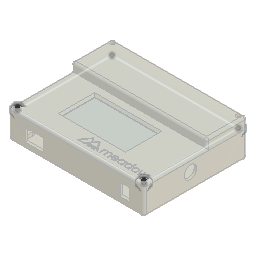
GNSS_Tracker_Enclosure (Autodesk Fusion 360 design; units mm, degrees)
Autodesk Fusion 360 part; units mm, degrees
(part 1 of 4)
sketch "Sketch1" plane through (0, 0, 0) normal (0, 0, 1) x (1, 0, 0) in component "GNSS_PCB"
  line L0 (50, 37.5) -> (-50, 37.5)
  line L1 (-50, 37.5) -> (-50, -37.5)
  line L2 (-50, -37.5) -> (50, -37.5)
  line L3 (50, -37.5) -> (50, 37.5)
  line L4 (50, 37.5) -> (-50, -37.5) construction
  line L5 (-50, 37.5) -> (50, -37.5) construction
  line L6 (0, 37.5) -> (0, -37.5) construction
  line L7 (-50, 0) -> (50, 0) construction
  line L8 (-30.5, 8.425) -> (30.5, 8.425)
  line L9 (30.5, 8.425) -> (30.5, -31.075)
  line L10 (30.5, -31.075) -> (-30.5, -31.075)
  line L11 (-30.5, -31.075) -> (-30.5, 8.425)
  line L12 (-27.5, 1.425) -> (22, 1.425)
  line L13 (22, 1.425) -> (22, -24.075)
  line L14 (22, -24.075) -> (-27.5, -24.075)
  line L15 (-27.5, -24.075) -> (-27.5, 1.425)
  line L16 (-38.5, 35.825) -> (38.5, 35.825)
  line L17 (38.5, 35.825) -> (38.5, 15.175)
  line L18 (38.5, 15.175) -> (-38.5, 15.175)
  line L19 (-38.5, 15.175) -> (-38.5, 35.825)
  line L20 (-33, -37.5) -> (-33, 37.5) construction
  line L21 (38, -37.5) -> (38, 37.5) construction
  line L22 (-28.5, -30.1) -> (-37.5, -30.1)
  line L23 (-37.5, -30.1) -> (-37.5, -37.5)
  line L24 (-37.5, -37.5) -> (-28.5, -37.5)
  line L25 (-28.5, -37.5) -> (-28.5, -30.1)
  line L26 (-28.5, -30.1) -> (-37.5, -37.5) construction
  line L27 (-37.5, -30.1) -> (-28.5, -37.5) construction
  line L28 (40.75, -28.5) -> (35.25, -28.5)
  line L29 (35.25, -28.5) -> (35.25, -40.5)
  line L30 (35.25, -40.5) -> (40.75, -40.5)
  line L31 (40.75, -40.5) -> (40.75, -28.5)
  line L32 (40.75, -28.5) -> (35.25, -40.5) construction
  line L33 (35.25, -28.5) -> (40.75, -40.5) construction
  line L34 (50, -4) -> (-50, -4) construction
  line L35 (-30.5, 3.275) -> (30.5, 3.275)
  line L36 (30.5, 3.275) -> (30.5, -25.925)
  line L37 (30.5, -25.925) -> (-30.5, -25.925)
  line L38 (-30.5, -25.925) -> (-30.5, 3.275)
  line L39 (-50, 35) -> (50, 35) construction
  line L40 (47.5, 37.5) -> (47.5, -37.5) construction
  line L41 (50, -35) -> (-50, -35) construction
  line L42 (-47.5, 37.5) -> (-47.5, -37.5) construction
  line L43 (45, 37.5) -> (45, -37.5) construction
  line L44 (-50, -32.5) -> (50, -32.5) construction
  line L45 (-50, 32.5) -> (50, 32.5) construction
  line L46 (-45, 37.5) -> (-45, -37.5) construction
  line L47 (-50, 30) -> (50, 30) construction
  line L48 (42.5, 37.5) -> (42.5, -37.5) construction
  line L49 (-50, -30) -> (50, -30) construction
  line L50 (-42.5, 37.5) -> (-42.5, -37.5) construction
  arc A0 (-50, -30) -> (-47.5, -32.5) centre (-47.5, -30) ccw
  arc A1 (-45, -35) -> (-47.5, -32.5) centre (-47.5, -35) ccw
  arc A2 (-45, -35) -> (-42.5, -37.5) centre (-42.5, -35) ccw
  arc A3 (47.5, -32.5) -> (50, -30) centre (47.5, -30) ccw
  arc A4 (47.5, -32.5) -> (45, -35) centre (47.5, -35) ccw
  arc A5 (42.5, -37.5) -> (45, -35) centre (42.5, -35) ccw
  arc A6 (50, 30) -> (47.5, 32.5) centre (47.5, 30) ccw
  arc A7 (45, 35) -> (47.5, 32.5) centre (47.5, 35) ccw
  arc A8 (45, 35) -> (42.5, 37.5) centre (42.5, 35) ccw
  arc A9 (-42.5, 37.5) -> (-45, 35) centre (-42.5, 35) ccw
  arc A10 (-47.5, 32.5) -> (-45, 35) centre (-47.5, 35) ccw
  arc A11 (-47.5, 32.5) -> (-50, 30) centre (-47.5, 30) ccw
  point P0 (-33, -33.8)
  point P1 (38, -34.5)
  point P2 (42.5, 35)
  point P3 (47.5, 30)
  point P4 (47.5, 35)
  point P5 (47.5, -30)
  point P6 (42.5, -35)
  point P7 (47.5, -35)
  point P8 (-47.5, 35)
  point P9 (-47.5, 30)
  point P10 (-42.5, 35)
  point P11 (-47.5, -35)
  point P12 (-47.5, -30)
  point P13 (-42.5, -35)
  point P14 (-50, -30)
  point P15 (-47.5, -32.5)
  point P16 (-45, -35)
  point P17 (-42.5, -37.5)
  dimension "d6" = 75
  dimension "d8" = 100
  dimension "d19" = 61
  dimension "d20" = 39.5
  dimension "d21" = 30.5
  dimension "d22" = 8.425
  dimension "d23" = 49.5
  dimension "d24" = 25.5
  dimension "d25" = 7
  dimension "d26" = 3
  dimension "d30" = 77
  dimension "d31" = 20.65
  dimension "d32" = 38.5
  dimension "d35" = 35.825
  dimension "d38" = 17
  dimension "d39" = 12
  dimension "d43" = 9
  dimension "d44" = 7.4
  dimension "d45" = 7.4
  dimension "d49" = 5.5
  dimension "d50" = 12
  dimension "d51" = 9
  dimension "d74" = 61
  dimension "d75" = 29.2
  dimension "d76" = 5.15
  dimension "d167" = 2.5
  dimension "d168" = 2.5
  dimension "d169" = 2.5
  dimension "d170" = 2.5
  dimension "d171" = 2.5
  dimension "d172" = 2.5
  dimension "d173" = 2.5
  dimension "d174" = 2.5
  dimension "d175" = 2.5
  dimension "d176" = 2.5
  dimension "d177" = 2.5
  dimension "d178" = 2.5
  constraint horizontal L0
  constraint perpendicular L0 L1
  constraint parallel L0 L2
  constraint parallel L1 L3
  constraint coincident L4 origin
  constraint coincident L5 origin
  constraint midpoint L0 L6.start
  constraint midpoint L2 L6.end
  constraint midpoint L1 L7.start
  constraint midpoint L3 L7.end
  constraint horizontal L8
  constraint vertical L9
  constraint horizontal L10
  constraint vertical L11
  constraint horizontal L12
  constraint vertical L13
  constraint horizontal L14
  constraint vertical L15
  constraint horizontal L16
  constraint vertical L17
  constraint horizontal L18
  constraint vertical L19
  constraint coincident L2 L20.start
  constraint coincident L0 L20.end
  constraint perpendicular L0 L20
  constraint coincident L2 L21.start
  constraint coincident L0 L21.end
  constraint perpendicular L0 L21
  constraint horizontal L22
  constraint perpendicular L22 L23
  constraint parallel L22 L24
  constraint parallel L23 L25
  constraint coincident L26 P0
  constraint coincident L27 P0
  constraint coincident L20 P0
  constraint horizontal L28
  constraint perpendicular L28 L29
  constraint parallel L28 L30
  constraint parallel L29 L31
  constraint coincident L32 P1
  constraint coincident L33 P1
  constraint coincident L21 P1
  constraint coincident L3 L34.start
  constraint coincident L1 L34.end
  constraint perpendicular L1 L34
  constraint horizontal L35
  constraint vertical L36
  constraint horizontal L37
  constraint vertical L38
  constraint coincident L11 L35.start
  constraint coincident L1 L39.start
  constraint coincident L3 L39.end
  constraint perpendicular L3 L39
  constraint coincident L0 L40.start
  constraint coincident L2 L40.end
  constraint perpendicular L2 L40
  constraint coincident L3 L41.start
  constraint coincident L1 L41.end
  constraint perpendicular L1 L41
  constraint coincident L0 L42.start
  constraint coincident L2 L42.end
  constraint perpendicular L2 L42
  constraint coincident L0 L43.start
  constraint coincident L2 L43.end
  constraint perpendicular L2 L43
  constraint coincident L1 L44.start
  constraint coincident L3 L44.end
  constraint perpendicular L3 L44
  constraint coincident L1 L45.start
  constraint coincident L3 L45.end
  constraint perpendicular L3 L45
  constraint coincident L0 L46.start
  constraint coincident L2 L46.end
  constraint perpendicular L2 L46
  constraint coincident L1 L47.start
  constraint coincident L3 L47.end
  constraint perpendicular L3 L47
  constraint coincident L0 L48.start
  constraint coincident L2 L48.end
  constraint perpendicular L2 L48
  constraint coincident L1 P14
  constraint coincident L3 L49.end
  constraint perpendicular L3 L49
  constraint coincident L0 L50.start
  constraint coincident L2 P17
  constraint perpendicular L2 L50
  constraint coincident L48 P2
  constraint coincident L39 P2
  constraint coincident L47 P3
  constraint coincident L40 P3
  constraint coincident L40 P4
  constraint coincident L39 P4
  constraint coincident L49 P5
  constraint coincident L40 P5
  constraint coincident L48 P6
  constraint coincident L41 P6
  constraint coincident L41 P7
  constraint coincident L40 P7
  constraint coincident L42 P8
  constraint coincident L39 P8
  constraint coincident L47 P9
  constraint coincident L42 P9
  constraint coincident L50 P10
  constraint coincident L39 P10
  constraint coincident L41 P11
  constraint coincident L42 P11
  constraint coincident L42 P12
  constraint coincident L49 P12
  constraint coincident L41 P13
  constraint coincident L50 P13
  constraint coincident P14 L49.start
  constraint coincident L42 P15
  constraint coincident L44 P15
  constraint coincident L46 P16
  constraint coincident L41 P16
  constraint coincident P17 L50.end
  constraint coincident P15 A0.end
  constraint coincident P16 A1.start
  constraint coincident L44 A3.start
  constraint coincident P5 A3.centre
  constraint coincident L43 A4.end
  constraint coincident P7 A4.centre
  constraint coincident L40 A6.end
  constraint coincident P3 A6.centre
  constraint coincident L43 A7.start
  constraint coincident P4 A7.centre
  constraint coincident L46 A9.end
  constraint coincident P10 A9.centre
  constraint coincident L45 A10.start
  constraint coincident P8 A10.centre
  measures "d6" distance of L0.end L1.end
  measures "d8" distance of L0.start L0.end
  measures "d19" distance of L8.start L8.end
  measures "d20" distance of L8.start L10.end
  measures "d21" distance of L6 L11
  measures "d22" distance of L7 L8
  measures "d23" distance of L12.start L12.end
  measures "d24" distance of L12.start L14.end
  measures "d25" distance of L8 L12
  measures "d26" distance of L11 L15
  measures "d30" distance of L16.start L16.end
  measures "d31" distance of L16.start L18.end
  measures "d32" distance of L6 L19
  measures "d35" distance of L7 L16
  measures "d38" distance of L1 L20
  measures "d39" distance of L3 L21
  measures "d43" distance of L23.end L24.end
  measures "d44" distance of L22.end L23.end
  measures "d45" distance of L2 L22
  measures "d49" distance of L29.end L30.end
  measures "d50" distance of L28.end L29.end
  measures "d51" distance of L2 L28
  measures "d74" distance of L35.start L35.end
  measures "d75" distance of L35.start L37.end
  measures "d76" distance of L8 L35
  measures "d167" distance of L0 L39
  measures "d168" distance of L3 L40
  measures "d169" distance of L1 L42
  measures "d170" distance of L2 L41
  measures "d171" distance of L42 L46
  measures "d172" distance of L39 L45
  measures "d173" distance of L40 L43
  measures "d174" distance of L41 L44
  measures "d175" distance of L43 L48
  measures "d176" distance of L45 L47
  measures "d177" distance of L44 L49
  measures "d178" distance of L46 L50
extrude "Extrude1" add sketch "Sketch1" along normal blind 1.7 contours L0 L1 L2 L3 L8 L9 L10 L11 L22 L23 L25 L28 L29 L31 L36 L38 A0 A1 A2 A3 A4 A5 A6 A7 A8 A9 A10 A11 | L2 L28 L29 L31 | L2 L10 L11 L22 L23 L24 L25 | L9 L10 L11 L22 L25 L37 | L10 L11 L22 L25 | L9 L11 L35 L36 L37 L38 | L8 L9 L11 L35 | L12 L13 L14 L15 | L16 L17 L18 L19 makes body 1 in component "GNSS_PCB"
sketch "Sketch2" plane through (0, 0, 1.7) normal (0, 0, 1) x (-1, 0, 0) in component "GNSS_PCB"
  line L0 (42.5, 37.5) -> (-42.5, 37.5)
  line L1 (-50, 30) -> (-50, -30)
  line L2 (-42.5, -37.5) -> (42.5, -37.5)
  line L3 (50, -30) -> (50, 30)
  line L4 (-35.25, 40.5) -> (-40.75, 40.5)
  line L5 (-35.25, 28.5) -> (-35.25, 40.5)
  line L6 (-40.75, 40.5) -> (-40.75, 28.5)
  line L7 (-38, 37.5) -> (-38, -37.5)
  line L8 (-38.5, -15.175) -> (38.5, -15.175)
  line L9 (-38.5, -35.825) -> (-38.5, -15.175)
  line L10 (38.5, -15.175) -> (38.5, -35.825)
  line L11 (38.5, -35.825) -> (-38.5, -35.825)
  line L12 (-40.75, 28.5) -> (-35.25, 28.5)
  arc A0 (-45, -35) -> (-42.5, -37.5) centre (-42.5, -35) ccw
  arc A1 (42.5, -37.5) -> (45, -35) centre (42.5, -35) ccw
  arc A2 (47.5, -32.5) -> (45, -35) centre (47.5, -35) ccw
  arc A3 (47.5, -32.5) -> (50, -30) centre (47.5, -30) ccw
  arc A4 (50, 30) -> (47.5, 32.5) centre (47.5, 30) ccw
  arc A5 (45, 35) -> (47.5, 32.5) centre (47.5, 35) ccw
  arc A6 (45, 35) -> (42.5, 37.5) centre (42.5, 35) ccw
  arc A7 (-42.5, 37.5) -> (-45, 35) centre (-42.5, 35) ccw
  arc A8 (-47.5, 32.5) -> (-45, 35) centre (-47.5, 35) ccw
  arc A9 (-47.5, 32.5) -> (-50, 30) centre (-47.5, 30) ccw
  arc A10 (-50, -30) -> (-47.5, -32.5) centre (-47.5, -30) ccw
  arc A11 (-45, -35) -> (-47.5, -32.5) centre (-47.5, -35) ccw
extrude "Extrude2" add sketch "Sketch2" along normal blind 18.5 separate body contours L7 L8 L10 L11 | L7 L8 L9 L11 makes body 2 in component "GNSS_PCB"
extrude "Extrude3" add sketch "Sketch2" along normal blind 7.5 separate body contours L0 L5 L7 L12 | L0 L4 L5 L6 | L0 L6 L7 L12 makes body 3 in component "GNSS_PCB"
fillet "Fillet1" radius 10.325 1 edges at (0, 15.175, 20.2) on bodies 2 in component "GNSS_PCB"
fillet "Fillet2" radius 10.325 1 edges at (0, 35.825, 20.2) on bodies 2 in component "GNSS_PCB"
ref_plane "WorkPlane1" through (36.625, -33, 3.6) normal (0, 0, 1) x (-1, 0, 0) in component "GNSS_PCB"
sketch "Sketch3" plane through (0, 0, 3.6) normal (0, 0, 1) x (1, 0, 0) in component "GNSS_PCB"
  line L0 (-28.5, -30.1) -> (-37.5, -30.1)
  line L1 (-37.5, -30.1) -> (-37.5, -37.5)
  line L2 (-28.5, -37.5) -> (-28.5, -30.1)
  line L3 (-50, -37.5) -> (50, -37.5)
extrude "Extrude4" add sketch "Sketch3" along normal blind 3.4 separate body makes body 4 in component "GNSS_PCB"
ref_plane "WorkPlane2" through (0, 0, 12.7) normal (0, 0, 1) x (-1, 0, 0) in component "GNSS_PCB"
sketch "Sketch4" plane through (0, 0, 12.7) normal (0, 0, 1) x (1, 0, 0) in component "GNSS_PCB"
  line L0 (-30.5, 8.425) -> (30.5, 8.425)
  line L1 (-30.5, -31.075) -> (-30.5, 8.425)
  line L2 (30.5, 8.425) -> (30.5, -31.075)
  line L3 (30.5, -31.075) -> (-30.5, -31.075)
extrude "Extrude5" add sketch "Sketch4" along normal blind 1.7 separate body makes body 5 in component "GNSS_PCB"
sketch "Sketch5" plane through (0, 0, 14.4) normal (0, 0, 1) x (-1, 0, 0) in component "GNSS_PCB"
  line L0 (-30.5, 31.075) -> (-30.5, -8.425)
  line L1 (-30.5, -8.425) -> (30.5, -8.425)
  line L2 (30.5, -8.425) -> (30.5, 31.075)
  line L3 (30.5, 31.075) -> (-30.5, 31.075)
sketch "Sketch6" plane through (0, 0, 14.4) normal (0, 0, 1) x (-1, 0, 0) in component "GNSS_PCB"
  line L0 (30.5, -3.275) -> (-30.5, -3.275)
  line L1 (-30.5, 25.925) -> (30.5, 25.925)
  line L2 (30.5, 25.925) -> (30.5, -3.275)
  line L3 (-30.5, -3.275) -> (-30.5, 25.925)
extrude "Extrude6" add sketch "Sketch6" along normal blind 1.3 separate body makes body 6 in component "GNSS_PCB"
sketch "Sketch7" plane through (0, 0, 15.7) normal (0, 0, 1) x (-1, 0, 0) in component "GNSS_PCB"
  line L0 (-30.5, -3.275) -> (30.5, -3.275)
  line L1 (30.5, -3.275) -> (30.5, 25.925)
  line L2 (30.5, 25.925) -> (-30.5, 25.925)
  line L3 (-30.5, 25.925) -> (-30.5, -3.275)
  line L4 (-22, 24.075) -> (27.5, 24.075)
  line L5 (-22, -1.425) -> (-22, 24.075)
  line L6 (27.5, 24.075) -> (27.5, -1.425)
  line L7 (27.5, -1.425) -> (-22, -1.425)
hole "Hole1" at (47.5, 30, 1.7) at (47.5, -30, 1.7) at (-47.5, 30, 1.7) at (-47.5, -30, 1.7) direction (0, 0, -1) diameter 2.1 end through all bodies 1 2 3 in component "GNSS_PCB"
ref_plane "WorkPlane1" through (0, 0, -3) normal (0, 0, 1) x (1, 0, 0) in component "GNSS_Enclosure_Bottom"
sketch "Sketch1 (2)" plane through (0, 0, -3) normal (0, 0, 1) x (1, 0, 0) in component "GNSS_Enclosure_Bottom"
  line L0 (-50, -37.5) -> (50, -37.5)
  line L1 (50, -37.5) -> (50, 37.5)
  line L2 (50, 37.5) -> (-50, 37.5)
  line L3 (-50, 37.5) -> (-50, -37.5)
  line L4 (51, -38.5) -> (51, 38.5)
  line L5 (51, 38.5) -> (-51, 38.5)
  line L6 (-51, 38.5) -> (-51, -38.5)
  line L7 (-51, -38.5) -> (51, -38.5)
  line L8 (-53, -40.5) -> (53, -40.5)
  line L9 (53, -40.5) -> (53, 40.5)
  line L10 (53, 40.5) -> (-53, 40.5)
  line L11 (-53, 40.5) -> (-53, -40.5)
  circle A0 centre (-47.5, 30) radius 1.05
  circle A1 centre (47.5, 30) radius 1.05
  circle A2 centre (47.5, -30) radius 1.05
  circle A3 centre (-47.5, -30) radius 1.05
  arc A4 (45, 35) -> (47.5, 32.5) centre (47.5, 35) ccw
  arc A5 (50, 30) -> (47.5, 32.5) centre (47.5, 30) ccw
  line L12 (50, -30) -> (50, 30)
  arc A6 (47.5, -32.5) -> (50, -30) centre (47.5, -30) ccw
  arc A7 (47.5, -32.5) -> (45, -35) centre (47.5, -35) ccw
  arc A8 (42.5, -37.5) -> (45, -35) centre (42.5, -35) ccw
  line L13 (-42.5, -37.5) -> (42.5, -37.5)
  arc A9 (-45, -35) -> (-42.5, -37.5) centre (-42.5, -35) ccw
  arc A10 (-45, -35) -> (-47.5, -32.5) centre (-47.5, -35) ccw
  arc A11 (-50, -30) -> (-47.5, -32.5) centre (-47.5, -30) ccw
  line L14 (-50, 30) -> (-50, -30)
  arc A12 (-47.5, 32.5) -> (-50, 30) centre (-47.5, 30) ccw
  arc A13 (-47.5, 32.5) -> (-45, 35) centre (-47.5, 35) ccw
  arc A14 (-42.5, 37.5) -> (-45, 35) centre (-42.5, 35) ccw
  line L15 (42.5, 37.5) -> (-42.5, 37.5)
  arc A15 (45, 35) -> (42.5, 37.5) centre (42.5, 35) ccw
  arc A16 (-47.5, 33.5) -> (-46, 35) centre (-47.5, 35) ccw
  arc A17 (-42.5, 38.5) -> (-46, 35) centre (-42.5, 35) ccw
  line L16 (42.5, 38.5) -> (-42.5, 38.5)
  arc A18 (46, 35) -> (42.5, 38.5) centre (42.5, 35) ccw
  arc A19 (46, 35) -> (47.5, 33.5) centre (47.5, 35) ccw
  arc A20 (51, 30) -> (47.5, 33.5) centre (47.5, 30) ccw
  line L17 (51, -30) -> (51, 30)
  arc A21 (47.5, -33.5) -> (51, -30) centre (47.5, -30) ccw
  arc A22 (47.5, -33.5) -> (46, -35) centre (47.5, -35) ccw
  arc A23 (42.5, -38.5) -> (46, -35) centre (42.5, -35) ccw
  line L18 (-42.5, -38.5) -> (42.5, -38.5)
  arc A24 (-46, -35) -> (-42.5, -38.5) centre (-42.5, -35) ccw
  arc A25 (-46, -35) -> (-47.5, -33.5) centre (-47.5, -35) ccw
  arc A26 (-51, -30) -> (-47.5, -33.5) centre (-47.5, -30) ccw
  line L19 (-51, 30) -> (-51, -30)
  arc A27 (-47.5, 33.5) -> (-51, 30) centre (-47.5, 30) ccw
  circle A28 centre (-47.5, 30) radius 3
  circle A29 centre (47.5, 30) radius 3
  circle A30 centre (-47.5, -30) radius 3
  circle A31 centre (47.5, -30) radius 3
  line L20 (-44.5, 30) -> (-44.5, 40.5)
  line L21 (-47.5, 27) -> (-53, 27)
  line L22 (-47.5, -27) -> (-53, -27)
  line L23 (-44.5, -30) -> (-44.5, -40.5)
  line L24 (47.5, -27) -> (53, -27)
  line L25 (44.5, -30) -> (44.5, -40.5)
  line L26 (47.5, 27) -> (53, 27)
  line L27 (44.5, 30) -> (44.5, 40.5)
  dimension "d87" = 1
  dimension "d88" = 3
  dimension "d192" = 1
  dimension "d193" = 6
  dimension "d194" = 6
  dimension "d195" = 6
  dimension "d196" = 6
  constraint concentric A0 A28
  constraint concentric A1 A29
  constraint concentric A3 A30
  constraint concentric A2 A31
  constraint coincident A28 L20.start
  constraint coincident L10 L20.end
  constraint tangent A28 L20
  constraint perpendicular L10 L20
  constraint coincident A28 L21.start
  constraint tangent A28 L21
  constraint perpendicular L11 L21
  constraint coincident A30 L22.start
  constraint tangent A30 L22
  constraint perpendicular L11 L22
  constraint coincident A30 L23.start
  constraint coincident L8 L23.end
  constraint tangent A30 L23
  constraint perpendicular L8 L23
  constraint coincident A31 L24.start
  constraint coincident L9 L24.end
  constraint tangent A31 L24
  constraint perpendicular L9 L24
  constraint coincident A31 L25.start
  constraint coincident L8 L25.end
  constraint tangent A31 L25
  constraint perpendicular L8 L25
  constraint coincident A29 L26.start
  constraint coincident L9 L26.end
  constraint tangent A29 L26
  constraint perpendicular L9 L26
  constraint coincident A29 L27.start
  constraint coincident L10 L27.end
  constraint tangent A29 L27
  constraint perpendicular L10 L27
  measures "d193" diameter of A28
  measures "d194" diameter of A29
  measures "d195" diameter of A30
  measures "d196" diameter of A31
extrude "Extrude1'" add sketch "Sketch1 (2)" against normal blind 2 separate body contours L0 L1 L2 L3 L12 A8 L13 A9 L14 A14 L15 A15 A28 A29 A30 A31 L20 L21 L22 L23 L24 L25 L26 L27 | L0 L7 L13 A23 L18 A24 L23 L25 | L0 A9 L23 | L0 A8 L25 | L0 A24 L23 | L0 L3 A9 A10 A24 A25 A26 A30 L23 | A9 A10 A30 L23 | L0 L1 A7 A8 A21 A22 A23 A31 L25 | L0 A23 L25 | A7 A8 A31 L25 | L0 L3 L6 L7 A24 A26 L23 | L0 L3 A24 A25 A26 | L7 A24 L23 | L3 A10 A11 L14 A30 | L0 L1 A21 A22 A23 | L0 L1 L4 L7 A21 A23 L25 | L7 A23 L25 | L1 L12 A6 A7 A31 | L7 L8 L18 L23 L25 | L6 L7 L8 L11 L19 L22 L23 | L3 A10 A11 A30 | L3 L14 A30 L22 | L4 L7 L8 L9 L17 L24 L25 | L1 A6 A7 A31 | L1 L12 A31 L24 | L3 L6 L14 A26 L19 A30 L22 | L3 L14 A30 | L3 L6 L14 L19 L21 L22 | L1 L4 L12 L17 A21 A31 L24 | L1 L12 A31 | L1 L4 L12 L17 L24 L26 | L3 L6 L14 L19 A27 A28 L21 | L3 L14 A28 L21 | L6 L11 L19 L21 L22 | L1 L12 A29 L26 | L1 L4 L12 A20 L17 A29 L26 | L4 L9 L17 L24 L26 | L3 L14 A28 | L3 L14 A12 A13 A28 | L5 L6 L10 L11 L19 L20 L21 | L1 A4 A5 L12 A29 | L1 L12 A29 | L4 L5 L9 L10 L17 L26 L27 | L3 A12 A13 A28 | L2 L3 A13 A14 A16 A17 A27 A28 L20 | A13 A14 A28 L20 | L2 L3 L5 L6 A17 A27 L20 | L1 A4 A5 A29 | A4 A15 A29 L27 | L1 L2 L4 L5 A18 A20 L27 | L2 L3 A16 A17 A27 | L2 A14 L20 | L1 L2 A4 A15 A18 A19 A20 A29 L27 | L2 A15 L27 | L1 L2 A18 A19 A20 | L5 L10 L16 L20 L27 | L2 L5 L15 A17 L16 A18 L20 L27 | L2 A17 L20 | L5 A17 L20 | L2 A18 L27 | L5 A18 L27 | A0 | A1 | A2 | A3 makes body 7 in component "GNSS_Enclosure_Bottom"
extrude "Extrude2'" add sketch "Sketch1 (2)" along normal up to surface (18.7 mm away) contours L7 L8 L18 L23 L25 | L6 L7 L8 L11 L19 L22 L23 | L4 L7 L8 L9 L17 L24 L25 | L6 L11 L19 L21 L22 | L4 L9 L17 L24 L26 | L5 L6 L10 L11 L19 L20 L21 | L4 L5 L9 L10 L17 L26 L27 | L5 L10 L16 L20 L27 bodies 7 in component "GNSS_Enclosure_Bottom"
extrude "Extrude10" add sketch "Sketch1 (2)" along normal up to surface (18.7 mm away) contours L0 L3 L6 L7 A24 A26 L23 | L0 L3 A24 A25 A26 | L7 A24 L23 | L0 L1 A21 A22 A23 | L0 L1 L4 L7 A21 A23 L25 | L7 A23 L25 | L2 L3 L5 L6 A17 A27 L20 | L1 L2 L4 L5 A18 A20 L27 | L2 L3 A16 A17 A27 | L1 L2 A18 A19 A20 | L5 A17 L20 | L5 A18 L27 bodies 7 in component "GNSS_Enclosure_Bottom"
extrude "Extrude11" add sketch "Sketch1 (2)" along normal blind 3 contours L0 A24 L23 | L0 L3 A9 A10 A24 A25 A26 A30 L23 | A9 A10 A30 L23 | L0 L1 A7 A8 A21 A22 A23 A31 L25 | L0 A23 L25 | A7 A8 A31 L25 | L3 A10 A11 L14 A30 | L1 L12 A6 A7 A31 | L3 A10 A11 A30 | L3 L14 A30 L22 | L1 A6 A7 A31 | L1 L12 A31 L24 | L3 L6 L14 A26 L19 A30 L22 | L3 L14 A30 | L1 L4 L12 L17 A21 A31 L24 | L1 L12 A31 | L3 L6 L14 L19 A27 A28 L21 | L3 L14 A28 L21 | L1 L12 A29 L26 | L1 L4 L12 A20 L17 A29 L26 | L3 L14 A28 | L3 L14 A12 A13 A28 | L1 A4 A5 L12 A29 | L1 L12 A29 | L3 A12 A13 A28 | L2 L3 A13 A14 A16 A17 A27 A28 L20 | A13 A14 A28 L20 | L1 A4 A5 A29 | A4 A15 A29 L27 | L1 L2 A4 A15 A18 A19 A20 A29 L27 | L2 A17 L20 | L2 A18 L27 | A0 | A1 | A2 | A3 bodies 7 in component "GNSS_Enclosure_Bottom"
sketch "Sketch7 (2)" plane through (0, 0, 0) normal (0, 0, 1) x (-1, 0, 0) in component "GNSS_Enclosure_Bottom"
  line L0 (44.5, -30) -> (44.5, -37.8723)
  arc A0 (44.5, -37.8723) -> (46, -35) centre (42.5, -35) ccw
  arc A1 (47.5, -33.5) -> (46, -35) centre (47.5, -35) ccw
  arc A2 (47.5, -33.5) -> (51, -30) centre (47.5, -30) ccw
  line L1 (51, -30) -> (51, -27)
  line L2 (51, -27) -> (47.5, -27)
  arc A3 (47.5, -27) -> (44.5, -30) centre (47.5, -30) ccw
  point P0 (47.5, -30)
  point P1 (47.5, 30)
  point P2 (-47.5, 30)
  point P3 (-47.5, -30)
sketch "Sketch3 (2)" plane through (0, -40.5, 0) normal (0, -1, 0) x (1, 0, 0) in component "GNSS_Enclosure_Bottom"
  line L0 (-53, 15.7) -> (-53, -5)
  line L1 (-53, -5) -> (53, -5)
  line L2 (53, -5) -> (53, 15.7)
  line L3 (53, 15.7) -> (-53, 15.7)
  line L4 (-37.5, 3.6) -> (-28.5, 3.6)
  line L5 (-28.5, 3.6) -> (-28.5, 7)
  line L6 (-28.5, 7) -> (-37.5, 7)
  line L7 (-37.5, 7) -> (-37.5, 3.6)
  line L8 (35.25, 1.7) -> (40.75, 1.7)
  line L9 (40.75, 1.7) -> (40.75, 9.2)
  line L10 (40.75, 9.2) -> (35.25, 9.2)
  line L11 (35.25, 9.2) -> (35.25, 1.7)
  line L12 (34.25, 10.2) -> (34.25, 0.7)
  line L13 (34.25, 0.7) -> (41.75, 0.7)
  line L14 (41.75, 0.7) -> (41.75, 10.2)
  line L15 (41.75, 10.2) -> (34.25, 10.2)
  line L16 (-33, 7) -> (-33, 3.6) construction
  line L17 (-37.5, 5.3) -> (-28.5, 5.3) construction
  line L18 (-26, 10.3) -> (-40, 10.3)
  line L19 (-40, 10.3) -> (-40, 0.3)
  line L20 (-40, 0.3) -> (-26, 0.3)
  line L21 (-26, 0.3) -> (-26, 10.3)
  line L22 (-26, 10.3) -> (-40, 0.3) construction
  line L23 (-40, 10.3) -> (-26, 0.3) construction
  point P0 (-33, 5.3)
  dimension "d102" = 1
  dimension "d107" = 14
  dimension "d108" = 10
  constraint midpoint L6 L16.start
  constraint midpoint L4 L16.end
  constraint midpoint L7 L17.start
  constraint midpoint L5 L17.end
  constraint horizontal L18
  constraint perpendicular L18 L19
  constraint parallel L18 L20
  constraint parallel L19 L21
  constraint coincident L22 P0
  constraint coincident L23 P0
  constraint midpoint L17 P0
  measures "d107" distance of L19.end L20.end
  measures "d108" distance of L18.end L19.end
extrude "Extrude4'" cut sketch "Sketch3 (2)" against normal up to surface (13.5 mm away) contours L8 L9 L10 L11 | L12 L13 L14 L15 bodies 7 in component "GNSS_Enclosure_Bottom"
extrude "Extrude5'" cut sketch "Sketch3 (2)" against normal up to surface (2 mm away) contours L4 L5 L6 L7 | L18 L19 L20 L21 bodies 7 in component "GNSS_Enclosure_Bottom"
sketch "Sketch1 (3)" plane through (0, 0, 15.7) normal (0, 0, 1) x (-1, 0, 0) in component "GNSS_Enclosure_Top"
  line L0 (-51, -30) -> (-51, 30)
  line L1 (-42.5, 38.5) -> (42.5, 38.5)
  line L2 (51, 30) -> (51, -30)
  line L3 (42.5, -38.5) -> (-42.5, -38.5)
  line L4 (-53, -40.5) -> (53, -40.5)
  line L5 (53, -40.5) -> (53, 40.5)
  line L6 (53, 40.5) -> (-53, 40.5)
  line L7 (-53, 40.5) -> (-53, -40.5)
  line L8 (-38.5, -35.825) -> (-38.5, -15.175)
  line L9 (38.5, -35.825) -> (-38.5, -35.825)
  line L10 (-38.5, -15.175) -> (38.5, -15.175)
  line L11 (38.5, -15.175) -> (38.5, -35.825)
  line L12 (53, -40.5) -> (-53, -40.5)
  line L13 (53, 40.5) -> (53, -40.5)
  line L14 (-53, -40.5) -> (-53, 40.5)
  line L15 (-53, 40.5) -> (53, 40.5)
  line L16 (53, -10.5) -> (-53, -10.5)
  line L17 (-51, 30) -> (-51, -30)
  line L18 (-42.5, -38.5) -> (42.5, -38.5)
  line L19 (51, -30) -> (51, 30)
  arc A0 (47.5, -33.5) -> (51, -30) centre (47.5, -30) ccw
  arc A1 (47.5, -33.5) -> (46, -35) centre (47.5, -35) ccw
  arc A2 (42.5, -38.5) -> (46, -35) centre (42.5, -35) ccw
  arc A3 (-46, -35) -> (-42.5, -38.5) centre (-42.5, -35) ccw
  arc A4 (-46, -35) -> (-47.5, -33.5) centre (-47.5, -35) ccw
  arc A5 (-51, -30) -> (-47.5, -33.5) centre (-47.5, -30) ccw
  arc A6 (-47.5, 33.5) -> (-51, 30) centre (-47.5, 30) ccw
  arc A7 (-47.5, 33.5) -> (-46, 35) centre (-47.5, 35) ccw
  arc A8 (-42.5, 38.5) -> (-46, 35) centre (-42.5, 35) ccw
  arc A9 (46, 35) -> (42.5, 38.5) centre (42.5, 35) ccw
  arc A10 (46, 35) -> (47.5, 33.5) centre (47.5, 35) ccw
  arc A11 (51, 30) -> (47.5, 33.5) centre (47.5, 30) ccw
  dimension "d111" = 4.675
  dimension "d112" = 4.675
  constraint coincident L13 L16.start
  constraint coincident L14 L16.end
  constraint perpendicular L14 L16
  measures "d111" distance of L4 L9
  measures "d112" distance of L10 L16
extrude "Extrude1''" add sketch "Sketch1 (3)" along normal blind 2 separate body contours L0 L2 L3 L4 L5 L7 L12 L13 L14 L16 L17 L18 L19 A0 A1 A2 A3 A4 A5 | L0 L1 L2 L5 L6 L7 L13 L14 L15 L16 L17 L19 A6 A7 A8 A9 A10 A11 | L0 L1 L2 L16 L17 L19 A6 A7 A8 A9 A10 A11 makes body 8 in component "GNSS_Enclosure_Top"
sketch "Sketch2 (2)" plane through (0, 0, 17.7) normal (0, 0, 1) x (-1, 0, 0) in component "GNSS_Enclosure_Top"
  line L0 (51, -10.5) -> (51, -30)
  line L1 (42.5, -38.5) -> (-42.5, -38.5)
  line L2 (-51, -30) -> (-51, -10.5)
  line L3 (-53, 40.5) -> (-53, -40.5)
  line L4 (-53, -40.5) -> (53, -40.5)
  line L5 (53, -40.5) -> (53, 40.5)
  line L6 (53, 40.5) -> (-53, 40.5)
  line L7 (-53, -8.5) -> (53, -8.5)
  arc A0 (47.5, -33.5) -> (51, -30) centre (47.5, -30) ccw
  arc A1 (47.5, -33.5) -> (46, -35) centre (47.5, -35) ccw
  arc A2 (42.5, -38.5) -> (46, -35) centre (42.5, -35) ccw
  arc A3 (-46, -35) -> (-42.5, -38.5) centre (-42.5, -35) ccw
  arc A4 (-46, -35) -> (-47.5, -33.5) centre (-47.5, -35) ccw
  arc A5 (-51, -30) -> (-47.5, -33.5) centre (-47.5, -30) ccw
  line L8 (-51, -10.5) -> (51, -10.5)
  constraint coincident L3 L7.start
  constraint coincident L5 L7.end
  constraint perpendicular L5 L7
sketch "Sketch3 (3)" plane through (53, 0, 0) normal (1, 0, 0) x (0, 1, 0) in component "GNSS_Enclosure_Top"
  line L0 (-40.5, 15.7) -> (40.5, 15.7)
  line L1 (40.5, 15.7) -> (40.5, 17.7)
  line L2 (40.5, 17.7) -> (-40.5, 17.7)
  line L3 (-40.5, 17.7) -> (-40.5, 15.7)
  arc A0 (35.825, 9.875) -> (15.175, 9.875) centre (25.5, 9.875) ccw
  line L4 (25.5, 20.2) -> (40.5, 20.2) construction
  line L5 (40.5, 20.2) -> (40.5, 17.7) construction
  line L6 (25.5, 22.2) -> (42.5, 22.2) construction
  line L7 (42.5, 22.2) -> (42.5, 17.7) construction
  constraint midpoint A0 L4.start
  constraint tangent A0 L4
  constraint perpendicular L1 L4
  constraint coincident L1.end L2.start
  constraint perpendicular L2 L5
extrude "Extrude2''" add sketch "Sketch2 (2)" along normal up to surface (4.5 mm away) contours L3 L4 L5 L7 bodies 8 in component "GNSS_Enclosure_Top"
sketch "Sketch4 (2)" plane through (0, 0, 22.2) normal (0, 0, 1) x (-1, 0, 0) in component "GNSS_Enclosure_Top"
  line L0 (42.5, -38.5) -> (-42.5, -38.5)
  line L1 (-51, -30) -> (-51, -10.5)
  line L2 (51, -10.5) -> (51, -30)
  line L3 (-53, -8.5) -> (-53, -40.5)
  line L4 (-53, -40.5) -> (53, -40.5)
  line L5 (53, -40.5) -> (53, -8.5)
  line L6 (53, -8.5) -> (-53, -8.5)
  arc A0 (47.5, -33.5) -> (51, -30) centre (47.5, -30) ccw
  arc A1 (47.5, -33.5) -> (46, -35) centre (47.5, -35) ccw
  arc A2 (42.5, -38.5) -> (46, -35) centre (42.5, -35) ccw
  arc A3 (-46, -35) -> (-42.5, -38.5) centre (-42.5, -35) ccw
  arc A4 (-46, -35) -> (-47.5, -33.5) centre (-47.5, -35) ccw
  arc A5 (-51, -30) -> (-47.5, -33.5) centre (-47.5, -30) ccw
  line L7 (-51, -10.5) -> (51, -10.5)
extrude "Extrude3'" add sketch "Sketch4 (2)" along normal blind 2 contours L0 L1 L2 A0 A1 A2 A3 A4 A5 L7 | L3 L4 L5 L6 bodies 8 in component "GNSS_Enclosure_Top"
sketch "Sketch4 (3)" plane through (53, 0, 0) normal (1, 0, 0) x (0, 1, 0) in component "GNSS_Enclosure_Bottom"
  line L0 (-40.5, 15.7) -> (-40.5, -5)
  line L1 (-40.5, -5) -> (40.5, -5)
  line L2 (40.5, -5) -> (40.5, 15.7)
  line L3 (40.5, 15.7) -> (-40.5, 15.7)
  line L4 (-4, 0) -> (-4, 15.7) construction
  point P0 (-4, 0)
  point P1 (-4, 8.2)
  dimension "d124" = 8.2
  constraint coincident P0 L4.start
  constraint coincident L3 L4.end
  constraint perpendicular L3 L4
  constraint coincident L4 P1
  measures "d124" distance of P0 P1
hole "Hole2" at (53, -4, 8.2) direction (-1, 0, 0) diameter 10 end up to surface (2 mm away) bodies 7 in component "GNSS_Enclosure_Bottom"
sketch "Sketch6 (2)" plane through (0, 0, 15.7) normal (0, 0, 1) x (-1, 0, 0) in component "GNSS_Enclosure_Bottom"
  line L0 (-51, -30) -> (-51, 30)
  line L1 (-42.5, 38.5) -> (42.5, 38.5)
  line L2 (51, 30) -> (51, -30)
  line L3 (42.5, -38.5) -> (-42.5, -38.5)
  line L4 (53, -40.5) -> (53, 40.5)
  line L5 (53, 40.5) -> (-53, 40.5)
  line L6 (-53, 40.5) -> (-53, -40.5)
  line L7 (-53, -40.5) -> (53, -40.5)
  arc A0 (47.5, -33.5) -> (51, -30) centre (47.5, -30) ccw
  arc A1 (47.5, -33.5) -> (46, -35) centre (47.5, -35) ccw
  arc A2 (42.5, -38.5) -> (46, -35) centre (42.5, -35) ccw
  arc A3 (-46, -35) -> (-42.5, -38.5) centre (-42.5, -35) ccw
  arc A4 (-46, -35) -> (-47.5, -33.5) centre (-47.5, -35) ccw
  arc A5 (-51, -30) -> (-47.5, -33.5) centre (-47.5, -30) ccw
  arc A6 (-47.5, 33.5) -> (-51, 30) centre (-47.5, 30) ccw
  arc A7 (-47.5, 33.5) -> (-46, 35) centre (-47.5, 35) ccw
  arc A8 (-42.5, 38.5) -> (-46, 35) centre (-42.5, 35) ccw
  arc A9 (46, 35) -> (42.5, 38.5) centre (42.5, 35) ccw
  arc A10 (46, 35) -> (47.5, 33.5) centre (47.5, 35) ccw
  arc A11 (51, 30) -> (47.5, 33.5) centre (47.5, 30) ccw
  point P0 (-53, -40.5)
  point P1 (53, -40.5)
sketch "Sketch5 (2)" plane through (0, 0, 15.7) normal (0, 0, -1) x (1, 0, 0) in component "GNSS_Enclosure_Top"
  line L0 (-51, -30) -> (-51, -10.5)
  line L1 (51, -10.5) -> (51, -30)
  line L2 (42.5, -38.5) -> (-42.5, -38.5)
  line L3 (53, -40.5) -> (53, 40.5)
  line L4 (53, 40.5) -> (-53, 40.5)
  line L5 (-53, 40.5) -> (-53, -40.5)
  line L6 (-53, -40.5) -> (53, -40.5)
  line L7 (51, -30) -> (51, 30)
  line L8 (42.5, 38.5) -> (-42.5, 38.5)
  line L9 (-51, 30) -> (-51, -30)
  line L10 (-42.5, -38.5) -> (42.5, -38.5)
  line L11 (-53, -40.5) -> (-53, 40.5)
  line L12 (-53, 40.5) -> (53, 40.5)
  line L13 (53, 40.5) -> (53, -40.5)
  line L14 (53, -40.5) -> (-53, -40.5)
  arc A0 (-51, -30) -> (-47.5, -33.5) centre (-47.5, -30) ccw
  arc A1 (47.5, -33.5) -> (51, -30) centre (47.5, -30) ccw
  arc A2 (47.5, -33.5) -> (46, -35) centre (47.5, -35) ccw
  arc A3 (42.5, -38.5) -> (46, -35) centre (42.5, -35) ccw
  arc A4 (-46, -35) -> (-42.5, -38.5) centre (-42.5, -35) ccw
  arc A5 (-46, -35) -> (-47.5, -33.5) centre (-47.5, -35) ccw
  arc A6 (-51, -30) -> (-47.5, -33.5) centre (-47.5, -30) ccw
  arc A7 (-46, -35) -> (-47.5, -33.5) centre (-47.5, -35) ccw
  arc A8 (-46, -35) -> (-42.5, -38.5) centre (-42.5, -35) ccw
  arc A9 (42.5, -38.5) -> (46, -35) centre (42.5, -35) ccw
  arc A10 (47.5, -33.5) -> (46, -35) centre (47.5, -35) ccw
  arc A11 (47.5, -33.5) -> (51, -30) centre (47.5, -30) ccw
  arc A12 (51, 30) -> (47.5, 33.5) centre (47.5, 30) ccw
  arc A13 (46, 35) -> (47.5, 33.5) centre (47.5, 35) ccw
  arc A14 (46, 35) -> (42.5, 38.5) centre (42.5, 35) ccw
  arc A15 (-42.5, 38.5) -> (-46, 35) centre (-42.5, 35) ccw
  arc A16 (-47.5, 33.5) -> (-46, 35) centre (-47.5, 35) ccw
  arc A17 (-47.5, 33.5) -> (-51, 30) centre (-47.5, 30) ccw
  line L15 (-51, -10.5) -> (51, -10.5)
sketch "Sketch6 (3)" plane through (0, 0, 15.7) normal (0, 0, 1) x (1, 0, 0) in component "GNSS_Enclosure_Top"
sketch "Sketch7 (3)" plane through (0, 0, 17.7) normal (0, 0, 1) x (-1, 0, 0) in component "GNSS_Enclosure_Top"
  line L0 (-53, -8.5) -> (53, -8.5)
  line L1 (53, -8.5) -> (53, 40.5)
  line L2 (53, 40.5) -> (-53, 40.5)
  line L3 (-53, 40.5) -> (-53, -8.5)
sketch "Sketch8" plane through (0, 0, 24.2) normal (0, 0, 1) x (-1, 0, 0) in component "GNSS_Enclosure_Top"
  line L0 (-53, -8.5) -> (-53, -40.5)
  line L1 (-53, -40.5) -> (53, -40.5)
  line L2 (53, -40.5) -> (53, -8.5)
  line L3 (53, -8.5) -> (-53, -8.5)
sketch "Sketch9" plane through (0, 0, 17.7) normal (0, 0, 1) x (-1, 0, 0) in component "GNSS_Enclosure_Top"
  line L0 (-53, -8.5) -> (53, -8.5)
  line L1 (53, -8.5) -> (53, 40.5)
  line L2 (53, 40.5) -> (-53, 40.5)
  line L3 (-53, 40.5) -> (-53, -8.5)
  line L4 (27.5, -1.425) -> (-22, -1.425)
  line L5 (27.5, 24.075) -> (27.5, -1.425)
  line L6 (-22, 24.075) -> (27.5, 24.075)
  line L7 (-22, -1.425) -> (-22, 24.075)
extrude "Extrude6'" cut sketch "Sketch9" against normal up to surface (2 mm away) contours L4 L5 L6 L7 bodies 8 in component "GNSS_Enclosure_Top"